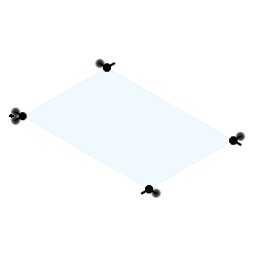
Printer_assembly (Autodesk Fusion 360 design; units mm, degrees)
Autodesk Fusion 360 part; units mm, degrees
note: some values were not read from the file. Set by a fixed rule: which sketch regions a step uses.
sketch "Sketch1" plane through (0, 0, 0) normal (0, 1, 0) x (1, 0, 0)
  line L0 (-300, -100) -> (600, -100)
  line L1 (600, -100) -> (600, 500)
  line L2 (600, 500) -> (-300, 500)
  line L3 (-300, 500) -> (-300, -100)
  constraint horizontal L0
  constraint vertical L1
  constraint horizontal L2
  constraint vertical L3
sketch "Sketch2" plane through (0, 0, 0) normal (0, 1, 0) x (1, 0, 0)
  line L0 (-280, -240) -> (-260, -240)
  line L1 (-260, -240) -> (-260, -260)
  line L2 (-260, -260) -> (-280, -260)
  line L3 (-280, -260) -> (-280, -240)
  circle A0 centre (-270, -250) radius 2.08
  line L4 (-270, -250) -> (-270, -253.9)
  line L5 (-270, -253.9) -> (-273.9, -253.9)
  line L6 (-273.9, -253.9) -> (-266.1, -253.9)
  line L7 (-266.1, -253.9) -> (-266.1, -246.1)
  line L8 (-266.1, -246.1) -> (-273.9, -246.1)
  line L9 (-273.9, -246.1) -> (-273.9, -253.9)
  line L10 (-270, -246.1) -> (-272.8, -246.1)
  line L11 (-270, -246.1) -> (-272.8, -246.1)
  line L12 (-266.1, -250) -> (-266.1, -247.2)
  line L13 (-266.1, -250) -> (-266.1, -252.8)
  line L14 (-270, -253.9) -> (-267.2, -253.9)
  line L15 (-270, -253.9) -> (-272.8, -253.9)
  line L16 (-273.9, -250) -> (-273.9, -252.8)
  line L17 (-273.9, -250) -> (-273.9, -247.2)
  line L18 (-270, -246.1) -> (-272.8, -246.1)
  line L19 (-270, -246.1) -> (-267, -246.1)
  line L20 (-266.1, -252.8) -> (-267.2, -253.9)
  line L21 (-266.1, -252.8) -> (-260, -258.9)
  line L22 (-267.2, -253.9) -> (-261.1, -260)
  line L23 (-267.2, -246.1) -> (-261.1, -240)
  line L24 (-266.1, -247.2) -> (-260, -241.1)
  line L25 (-267.2, -246.1) -> (-266.1, -247.2)
  line L26 (-273.9, -247.2) -> (-280, -241.1)
  line L27 (-272.8, -246.1) -> (-278.9, -240)
  line L28 (-273.9, -247.2) -> (-272.8, -246.1)
  line L29 (-272.8, -253.9) -> (-278.9, -260)
  line L30 (-273.9, -252.8) -> (-280, -258.9)
  line L31 (-272.8, -253.9) -> (-273.9, -252.8)
  line L32 (-270, -240) -> (-266.9, -240)
  line L33 (-270, -240) -> (-266.9, -240)
  line L34 (-266.9, -240) -> (-273.1, -240)
  line L35 (-280, -250) -> (-280, -244.55)
  line L36 (-280, -244.55) -> (-274.35, -244.55)
  line L37 (-270, -240) -> (-275.45, -240)
  line L38 (-275.45, -240) -> (-275.45, -244.55)
  line L39 (-280, -250) -> (-280, -255.45)
  line L40 (-280, -255.45) -> (-275.45, -255.45)
  line L41 (-275.45, -255.45) -> (-275.45, -260)
  line L42 (-270, -260) -> (-275.45, -260)
  line L43 (-270, -260) -> (-264.55, -260)
  line L44 (-264.55, -260) -> (-264.55, -255)
  line L45 (-260, -255.45) -> (-264.55, -255.45)
  line L46 (-264.55, -240) -> (-264.55, -245)
  line L47 (-260, -114.0508) -> (-264.55, -114.0508)
  line L48 (-260, -244.8999) -> (-265.9999, -244.8999)
  line L49 (-270, -240) -> (-273.1, -240)
  line L50 (-275.45, -240) -> (-275.45, -241)
  line L51 (-275.45, -241.6476) -> (-272.725, -241.6476)
  line L52 (-272.725, -241.6476) -> (-274, -240)
  line L53 (-280, -250) -> (-280, -246.9)
  line L54 (-275.45, -244.55) -> (-272.548, -244.55)
  line L55 (-275.45, -244.55) -> (-278.352, -244.55)
  line L56 (-278.352, -244.55) -> (-278.352, -246.9)
  line L57 (-278.352, -246.9) -> (-279.9723, -245.591)
  line L58 (-279.9723, -245.591) -> (-280, -244.55)
  line L59 (-275.45, -258.352) -> (-273.1, -258.352)
  line L60 (-273.1, -258.352) -> (-274.409, -259.9723)
  line L61 (-278.3524, -252.725) -> (-280, -254)
  line L62 (-278.3524, -255.45) -> (-278.3524, -252.725)
  line L63 (-261.648, -255.45) -> (-261.648, -253.1)
  line L64 (-261.648, -253.1) -> (-260.0277, -254.409)
  line L65 (-267.275, -258.3524) -> (-266, -260)
  line L66 (-264.55, -258.3524) -> (-267.275, -258.3524)
  line L67 (-264.55, -241.648) -> (-266.9, -241.648)
  line L68 (-266.9, -241.648) -> (-265.591, -240.0277)
  line L69 (-261.6476, -247.275) -> (-260, -246)
  line L70 (-261.6476, -244.55) -> (-261.6476, -247.275)
  line L71 (-274.409, -259.9723) -> (-275.45, -260)
  line L72 (-266, -260) -> (-264.55, -260)
  line L73 (-260.0277, -254.409) -> (-260, -255.45)
  line L74 (-260, -246) -> (-260, -244.8999)
  line L75 (-265.591, -240.0277) -> (-264.55, -240)
  line L76 (-280, -254) -> (-280, -255.45)
  line L77 (300, -500) -> (300, 100)
  line L78 (300, 100) -> (-600, 100)
  line L79 (-600, 100) -> (-600, -500)
  line L80 (-600, -500) -> (300, -500)
  dimension "d3" = 4.16
  dimension "d4" = 3.9
  dimension "d5" = 3.9
  dimension "d6" = 7.8
  dimension "d7" = 7.8
  dimension "d8" = 2.8
  dimension "d9" = 2.8
  dimension "d10" = 2.8
  dimension "d11" = 2.8
  dimension "d12" = 2.8
  dimension "d13" = 2.8
  dimension "d14" = 2.8
  dimension "d15" = 2.8
  dimension "d17" = 360
  dimension "d18" = 3.1
  dimension "d19" = 3.1
  dimension "d20" = 6.2
  dimension "d21" = 5.45
  dimension "d22" = 5.45
  dimension "d23" = 5.45
  dimension "d24" = 5.45
  dimension "d25" = 5.45
  dimension "d26" = 3.1
  dimension "d27" = 3.1
  dimension "d28" = 2.902
  dimension "d29" = 2.902
  dimension "d30" = 2.083
  dimension "d32" = 360
  constraint horizontal L0
  constraint perpendicular L0 L1
  constraint perpendicular L1 L2
  constraint perpendicular L0 L3
  constraint coincident A0.centre L4.start
  constraint vertical L4
  constraint perpendicular L4 L5
  constraint parallel L5 L6
  constraint perpendicular L5 L7
  constraint perpendicular L7 L8
  constraint perpendicular L6 L9
  constraint midpoint L8 L10.start
  constraint coincident L8 L10.end
  constraint midpoint L7 L12.start
  constraint perpendicular L8 L12
  constraint perpendicular L6 L13
  constraint perpendicular L7 L14
  constraint perpendicular L4 L15
  constraint midpoint L9 L16.start
  constraint perpendicular L6 L16
  constraint parallel L9 L17
  constraint coincident L8 L19.end
  constraint perpendicular L7 L19
  constraint coincident L1 L21.end
  constraint perpendicular L20 L21
  constraint coincident L2 L22.end
  constraint perpendicular L20 L22
  constraint midpoint L0 L32.start
  constraint coincident L0 L32.end
  constraint perpendicular L1 L33
  constraint parallel L0 L34
  constraint midpoint L3 L35.start
  constraint coincident L3 L35.end
  constraint coincident L27 L36.end
  constraint perpendicular L3 L36
  constraint parallel L0 L37
  constraint coincident L36 L38.end
  constraint perpendicular L36 L38
  constraint parallel L3 L39
  constraint perpendicular L3 L40
  constraint coincident L2 L41.end
  constraint perpendicular L2 L41
  constraint midpoint L2 L42.start
  constraint parallel L2 L43
  constraint perpendicular L43 L44
  constraint coincident L1 L45.start
  constraint coincident L44 L45.end
  constraint perpendicular L44 L45
  constraint coincident L0 L46.start
  constraint perpendicular L0 L46
  constraint coincident L1 L47.start
  constraint coincident L46 L47.end
  constraint perpendicular L46 L47
  constraint coincident L1 L48.start
  constraint coincident L23 L48.end
  constraint perpendicular L46 L48
  constraint parallel L37 L49
  constraint coincident L38 L50.end
  constraint perpendicular L37 L50
  constraint coincident L38 L51.start
  constraint perpendicular L38 L51
  constraint coincident L0 L52.end
  constraint coincident L3 L53.end
  constraint coincident L36 L54.end
  constraint perpendicular L38 L55
  constraint perpendicular L55 L56
  measures "d3" diameter of A0
  measures "d4" distance of A0.centre L4.end
  measures "d5" distance of L4.end L5.end
  measures "d6" distance of L5.end L6.end
  measures "d7" distance of L6.end L7.end
  measures "d8" distance of L10.start L10.end
  measures "d9" distance of L10.start L10.end
  measures "d10" distance of L12.start L12.end
  measures "d11" distance of L12.start L13.end
  measures "d12" distance of L4.end L14.end
  measures "d13" distance of L4.end L15.end
  measures "d14" distance of L16.start L16.end
  measures "d15" distance of L16.start L17.end
  measures "d18" distance of L32.start L32.end
  measures "d19" distance of L32.start L32.end
  measures "d20" distance of L32.end L34.end
  measures "d21" distance of L35.start L35.end
  measures "d22" distance of L32.start L37.end
  measures "d23" distance of L35.start L39.end
  measures "d24" distance of L42.start L41.end
  measures "d25" distance of L42.start L43.end
  measures "d26" distance of L32.start L34.end
  measures "d27" distance of L35.start L53.end
  measures "d28" distance of L38.end L54.end
  measures "d29" distance of L38.end L55.end
  measures "d30" distance of L56.end L57.end
extrude "Extrude2" add sketch "Sketch2" along normal blind 7 contours L0 L3 L26 L27 L36 L38 L55 | L0 L27 L38 L50 | L3 L26 L36 L55 | L0 L37 L38 L50 L51 L52 | L27 L36 L38 L54 | L36 L56 L57 L58 | L8 L9 L26 L27 L36 L54 L55 | L5 L6 L7 L8 L9 L10 L11 L12 L13 L14 L15 L16 L17 L18 L19 L20 L25 L28 L31 | L8 L9 L28 | L3 L39 L40 L61 L62 L76 | L5 L6 L9 L31 | L5 L6 L9 L29 L30 L40 L41 | L7 L8 L19 L23 L24 L48 | L7 L8 L19 L25 | L3 L30 L40 | L2 L3 L29 L30 L40 L41 | L0 L23 L46 | L46 L67 L68 L75 | L23 L46 L48 | L2 L29 L41 | L0 L1 L23 L24 L46 L48 | L1 L24 L48 | L6 L7 L20 | L6 L7 L21 L22 L44 L45 | L41 L59 L60 L71 | L1 L48 L69 L70 L74 | L1 L2 L21 L22 L44 L45 | L2 L22 L44 | L1 L21 L45 | L2 L43 L44 L65 L66 L72 | L45 L63 L64 L73
chamfer "Chamfer1" distance 0.2 angle 45 8 edges at (-273.1, 3.5, 258.352) (-272.725, 3.5, 241.6476) (-278.352, 3.5, 246.9) (-278.3524, 3.5, 252.725) (-261.6476, 3.5, 247.275) (-266.9, 3.5, 241.648) (-261.648, 3.5, 253.1) (-267.275, 3.5, 258.3524)
fillet "Fillet1" radius 1 4 edges at (-280, 3.5, 260) (-260, 3.5, 260) (-280, 3.5, 240) (-260, 3.5, 240)
sketch "Sketch3" plane through (0, 1, 0) normal (0, 1, 0) x (-1, 0, 0)
  line L0 (300, -500) -> (300, 100)
  line L1 (300, 100) -> (-600, 100)
  line L2 (-600, 100) -> (-600, -500)
  line L3 (-600, -500) -> (300, -500)
  line L4 (300, -500) -> (300, -550)
  line L5 (300, -550) -> (300, -500)
  line L6 (300, -500) -> (350, -500)
  line L7 (300, 100) -> (350, 100)
  line L8 (300, 100) -> (300, 150)
  line L9 (-600, 100) -> (-600, 150)
  line L10 (-600, 150) -> (-600, 100)
  line L11 (-600, 100) -> (-650, 100)
  line L12 (-600, -500) -> (-650, -500)
  line L13 (-650, -500) -> (-600, -500)
  line L14 (-600, -500) -> (-600, -550)
  dimension "d39" = 50
  dimension "d40" = 50
  dimension "d41" = 50
  dimension "d42" = 50
  dimension "d43" = 50
  dimension "d44" = 50
  dimension "d45" = 50
  dimension "d46" = 50
  constraint coincident L0.start L3.end
  constraint perpendicular L3 L4
  constraint perpendicular L0 L6
  constraint coincident L0.end L1.start
  constraint perpendicular L0 L7
  constraint perpendicular L7 L8
  constraint coincident L1.end L2.start
  constraint perpendicular L1 L9
  constraint perpendicular L10 L11
  constraint coincident L2.end L3.start
  constraint perpendicular L2 L12
  constraint perpendicular L12 L14
  measures "d39" distance of L0.start L4.end
  measures "d40" distance of L0.start L6.end
  measures "d41" distance of L0.end L7.end
  measures "d42" distance of L0.end L8.end
  measures "d43" distance of L1.end L9.end
  measures "d44" distance of L1.end L11.end
  measures "d45" distance of L2.end L12.end
  measures "d46" distance of L2.end L14.end
move_body "Move3" bodies 1 to x (1, 0, 0) y (0, 1, 0) z (0, 0, 1) at (-70, 0, -110)
